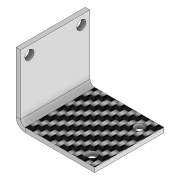
# Autodesk Inventor part: Clamps
Saved by Autodesk Inventor 2021 (Build 250183000, 183)
## iProperties
Created: 2021-07-10
Part Number: Clamps
Material: Generic
Document SubType Name: Sheet Metal
Designer: RahulRC
Density: 1 g/cm^3
Sheet Metal Rule: Default_mm
Appearance: Default
Author: RahulRC
Autodesk Inventor part; units mm, degrees
ref_plane "YZ Plane" through (0, 0, 0) normal (1, 0, 0) x (0, 1, 0)
ref_plane "XZ Plane" through (0, 0, 0) normal (0, 1, 0) x (-1, 0, 0)
ref_plane "XY Plane" through (0, 0, 0) normal (0, 0, 1) x (1, 0, 0)
sketch "Sketch1" plane through (0, 0, 0) normal (0, 1, 0) x (-1, 0, 0)
  line L0 (0, 0) -> (-15, 0)
  line L1 (-15, 0) -> (-15, -15)
  line L2 (-15, -15) -> (0, -15)
  line L3 (0, -15) -> (0, 0)
extrude "Plate1" add sketch "Sketch1" along normal blind 1
sketch "Sketch2" plane through (1, 0, 0) normal (-1, 0, 0) x (0, -1, 0)
  line L0 (0, -15) -> (0, 0)
  line L1 (0, 0) -> (-17, 0)
  line L2 (-17, 0) -> (-17, -15)
  line L3 (-17, -15) -> (0, -15)
  constraints: 6 end point, 1 horizontal, 1 perpendicular, 1 vertical
edge flange "Flange1" height 17 angle 90 thickness 1 bend radius 1 thickness toward (-1, 0, 0) relief tear relief width 1 relief depth 0.5 edges at (0, 1, -7.5) wall of the first edge with corners at (1, 0, -15) (1, 0, 0) (1, 17, 0) (1, 17, -15)
bend "Bend1"
corner "Corner1"
sketch "Sketch3" plane through (0, 1, 0) normal (0, 1, 0) x (1, 0, 0)
  circle A0 centre (13.1306, 13.1131) radius 1
  line L0 (2, 15) -> (15, 15) projected
  circle A1 centre (13.1306, 1.887) radius 1
  point P0 (0, 0)
  constraints: 2 centre point
extrude "Extrusion1" cut sketch "Sketch3" against normal through all
sketch "Sketch4" plane through (1, 17, 0) normal (1, 0, 0) x (0, 0, -1)
  circle A0 centre (2.6622, -2.6905) radius 1
  circle A1 centre (12.8576, -2.6905) radius 1
  point P0 (0, -17)
  constraints: 2 centre point
extrude "Extrusion2" cut sketch "Sketch4" against normal blind 10
equation "\"d2\" = Thickness"
equation "\"d3\" = BendReliefWidth"
equation "\"d4\" = BendReliefDepth"
equation "\"d5\" = MinimumRemnant"
equation "\"d6\" = TransitionRadius"
equation "\"d9\" = BendRadius"
equation "\"d10\" = CornerReliefSize"
equation "\"d11\" = GapSize"
equation "\"d12\" = JacobiRadiusSize"
equation "\"BendRadius\" = Thickness"
equation "\"BendReliefWidth\" = Thickness"
equation "\"BendReliefDepth\" = 0.5 * Thickness"
equation "\"CornerReliefSize\" = 4 * Thickness"
equation "\"MinimumRemnant\" = 2 * Thickness"
equation "\"TransitionRadius\" = BendRadius"
equation "\"JacobiRadiusSize\" = BendRadius"
equation "\"GapSize\" = Thickness"
equation "\"Thickness\" = 1"
body "Solid1"
